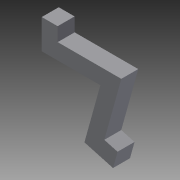
# Autodesk Inventor part: AcutePlateAttacher_v1
Saved by Autodesk Inventor 2013 (Build 170138000, 138)
## iProperties
Created: 2013-01-17
Part Number: AcutePlateAttacher_v1
Material: Generic
Document SubType Name: Modeling
Designer: motoennies
Density: 1 g/cm^3
Author: motoennies
Autodesk Inventor part; units mm, degrees
ref_plane "YZ Plane" through (0, 0, 0) normal (1, 0, 0) x (0, 1, 0)
ref_plane "XZ Plane" through (0, 0, 0) normal (0, 1, 0) x (-1, 0, 0)
ref_plane "XY Plane" through (0, 0, 0) normal (0, 0, 1) x (1, 0, 0)
sketch "Sketch1" plane through (0, 0, 0) normal (0, 0, 1) x (1, 0, 0)
  line L0 (0, 0) -> (0, 17.78)
  line L1 (0, 17.78) -> (9.525, 17.78)
  line L2 (9.525, 17.78) -> (9.525, 9.525)
  line L3 (9.525, 9.525) -> (47.625, 9.525)
  line L4 (47.625, 9.525) -> (37.4432, -27.1893)
  line L5 (37.4432, -27.1893) -> (45.398, -29.3954)
  line L6 (45.398, -29.3954) -> (42.6828, -39.1859)
  line L7 (42.6828, -39.1859) -> (25.5495, -34.4344)
  line L8 (25.5495, -34.4344) -> (35.099, 0)
  line L9 (35.099, 0) -> (0, 0)
  dimension "d7" = 17.78
  dimension "d8" = 9.525
  dimension "d9" = 8.255
  dimension "d10" = 38.1
  dimension "d11" = 38.1
  dimension "d12" = 74.5
  dimension "d13" = 8.255
  dimension "d14" = 10.16
  dimension "d15" = 17.78
  constraints: 20 end point, 5 perpendicular, 3 parallel, 1 vertical
  measures "d7" distance of L0.start L0.end
  measures "d8" distance of L0.end L1.end
  measures "d9" distance of L1.end L2.end
  measures "d10" distance of L2.end L3.end
  measures "d11" distance of L3.end L4.end
  measures "d12" angle of L3 L4
  measures "d13" distance of L4.end L5.end
  measures "d14" distance of L5.end L6.end
  measures "d15" distance of L6.end L7.end
extrude "Extrusion1" add sketch "Sketch1" along normal blind 10.16
body "Solid1"
